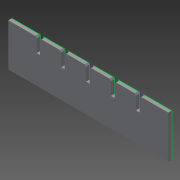
# Autodesk Inventor part: SlotRuler
Saved by Autodesk Inventor 2015 (Build 190159000, 159)
## iProperties
Created: 2015-02-15
Part Number: SlotRuler
Material: Generic
Document SubType Name: Modeling
Designer: Iain
Density: 1 g/cm^3
Appearance: Default
Author: Iain
Autodesk Inventor part; units mm, degrees
ref_plane "YZ Plane" through (0, 0, 0) normal (1, 0, 0) x (0, 1, 0)
ref_plane "XZ Plane" through (0, 0, 0) normal (0, 1, 0) x (-1, 0, 0)
ref_plane "XY Plane" through (0, 0, 0) normal (0, 0, 1) x (1, 0, 0)
sketch "Sketch1" plane through (0, 0, 0) normal (0, 1, 0) x (-1, 0, 0)
  line L0 (75, -15) -> (-75, -15)
  line L1 (-75, -15) -> (-75, 15)
  line L2 (-75, 15) -> (75, 15)
  line L3 (75, 15) -> (75, -15)
  point P0 (0, 0)
  point P1 (0, -15)
  point P2 (75, 0)
  point P3 (0, 15)
  dimension "d0" = 150
  dimension "d1" = 30
  constraints: 8 end point, 3 midpoint, 2 parallel, 1 horizontal, 1 horizontal alignment, 1 perpendicular, 1 vertical alignment
  measures "d0" distance of L1.end L2.end
  measures "d1" distance of L2.end L0.start
extrude "Extrusion1" add sketch "Sketch1" along normal blind 2.5
sketch "Sketch3" plane through (0, 2.5, 0) normal (0, 1, 0) x (1, 0, 0)
  line L0 (-75, 15) -> (-75, -15) projected
  line L1 (-75, -15) -> (75, -15) projected
  line L2 (-55, -15) -> (-52.7, -15)
  line L3 (-52.7, -15) -> (-52.7, -5)
  line L4 (-52.7, -5) -> (-55, -5)
  line L5 (-55, -5) -> (-55, -15)
  point P0 (0, 0)
  point P1 (-53.85, -15)
  point P2 (0, -15)
  dimension "d4" = 2.3
  dimension "d5" = 10
  dimension "d6" = 20
  constraints: 8 end point, 2 midpoint, 2 parallel, 1 horizontal, 1 horizontal alignment, 1 perpendicular
  measures "d4" distance of L3.end L4.end
  measures "d5" distance of L4.end L2.start
  measures "d6" distance from line of L0 L4.end
extrude "-0.2" cut sketch "Sketch3" along normal through all both and the other way through all
sketch "Sketch4" plane through (0, 2.5, 0) normal (0, 1, 0) x (1, 0, 0)
  line L0 (-75, -15) -> (-55, -15) projected
  line L1 (-37.7, -5) -> (-35.3, -5)
  line L2 (-35.3, -5) -> (-35.3, -15)
  line L3 (-35.3, -15) -> (-37.7, -15)
  line L4 (-37.7, -15) -> (-37.7, -5)
  point P0 (-52.7, -15)
  point P1 (0, 0)
  point P2 (-36.5, -15)
  point P3 (-65, -15)
  dimension "d9" = 10
  dimension "d10" = 2.4
  dimension "d11" = 15
  constraints: 8 end point, 2 midpoint, 2 parallel, 1 horizontal, 1 horizontal alignment, 1 perpendicular
  measures "d9" distance of L3.end L1.start
  measures "d10" distance of L1.start L1.end
  measures "d11" distance of point (-52.7, -15) L3.end
extrude "-0.1" cut sketch "Sketch4" against normal through all
sketch "Sketch5" plane through (0, 2.5, 0) normal (0, 1, 0) x (1, 0, 0)
  line L0 (-75, -15) -> (-55, -15) projected
  line L1 (-20.3, -5) -> (-17.8, -5)
  line L2 (-17.8, -5) -> (-17.8, -15)
  line L3 (-17.8, -15) -> (-20.3, -15)
  line L4 (-20.3, -15) -> (-20.3, -5)
  point P0 (-35.3, -5)
  point P1 (0, 0)
  point P2 (-19.05, -15)
  point P3 (-65, -15)
  dimension "d15" = 10
  dimension "d16" = 2.5
  dimension "d17" = 15
  constraints: 8 end point, 2 midpoint, 2 parallel, 1 horizontal, 1 horizontal alignment, 1 perpendicular
  measures "d15" distance of L1.end L2.end
  measures "d16" distance of L1.start L1.end
  measures "d17" distance of point (-35.3, -5) L1.start
extrude "0.0" cut sketch "Sketch5" against normal through all
sketch "Sketch6" plane through (0, 2.5, 0) normal (0, 1, 0) x (1, 0, 0)
  line L0 (-75, -15) -> (-55, -15) projected
  line L1 (-2.8, -15) -> (-0.2, -15)
  line L2 (-0.2, -15) -> (-0.2, -5)
  line L3 (-0.2, -5) -> (-2.8, -5)
  line L4 (-2.8, -5) -> (-2.8, -15)
  point P0 (-17.8, -5)
  point P1 (0, 0)
  point P2 (-1.5, -15)
  point P3 (-65, -15)
  dimension "d20" = 10
  dimension "d21" = 2.6
  dimension "d22" = 15
  constraints: 8 end point, 2 midpoint, 2 parallel, 1 horizontal, 1 horizontal alignment, 1 perpendicular
  measures "d20" distance of L1.end L2.end
  measures "d21" distance of L2.end L3.end
  measures "d22" distance of point (-17.8, -5) L3.end
extrude "+0.1" cut sketch "Sketch6" against normal through all
sketch "Sketch7" plane through (0, 2.5, 0) normal (0, 1, 0) x (1, 0, 0)
  line L0 (-75, -15) -> (-55, -15) projected
  line L1 (14.8, -15) -> (17.5, -15)
  line L2 (17.5, -15) -> (17.5, -5)
  line L3 (17.5, -5) -> (14.8, -5)
  line L4 (14.8, -5) -> (14.8, -15)
  point P0 (-0.2, -5)
  point P1 (0, 0)
  point P2 (16.15, -15)
  point P3 (-65, -15)
  dimension "d25" = 10
  dimension "d26" = 2.7
  dimension "d27" = 15
  constraints: 8 end point, 2 midpoint, 2 parallel, 1 horizontal, 1 horizontal alignment, 1 perpendicular
  measures "d25" distance of L1.end L2.end
  measures "d26" distance of L2.end L3.end
  measures "d27" distance of point (-0.2, -5) L3.end
extrude "+0.2" cut sketch "Sketch7" against normal through all
sketch "Sketch8" plane through (0, 2.5, 0) normal (0, 1, 0) x (1, 0, 0)
  line L0 (75, 15) -> (-75, 15) projected
  line L1 (-75, 15) -> (-75, -15) projected
  line L2 (-75, -15) -> (-55, -15) projected
  line L3 (-75, 15) -> (37.5, 15)
  line L4 (37.5, 15) -> (37.5, -15)
  line L5 (37.5, -15) -> (-75, -15)
  line L6 (-75, -15) -> (-75, 15)
  point P0 (17.5, -5)
  point P1 (0, 0)
  point P2 (-18.75, -15)
  point P3 (-65, -15)
  point P4 (-18.75, 15)
  point P5 (0, 15)
  point P6 (-75, 0)
  point P7 (-75, 0)
  dimension "d30" = 20
  constraints: 8 end point, 6 midpoint, 2 horizontal alignment, 2 parallel, 1 coincident, 1 horizontal, 1 perpendicular
  measures "d30" distance from line of L4 point (17.5, -5)
extrude "Extrusion7" cut sketch "Sketch8" against normal through all keep common part
sketch "Sketch9" plane through (0, 2.5, 0) normal (0, 1, 0) x (1, 0, 0)
  line L0 (37.5, 15) -> (37.5, -15) projected
  line L1 (37.5, 15) -> (-75, 15) projected
  line L2 (-75, 15) -> (-75, -15) projected
  line L3 (-75, -15) -> (-55, -15) projected
  line L4 (-55, -15) -> (-55, -5) projected
  line L5 (-55, -5) -> (-52.7, -5) projected
  line L6 (-52.7, -5) -> (-52.7, -15) projected
  line L7 (-52.7, -15) -> (-37.7, -15) projected
  line L8 (-37.7, -15) -> (-37.7, -5) projected
  line L9 (-37.7, -5) -> (-35.3, -5) projected
  line L10 (-35.3, -5) -> (-35.3, -15) projected
  line L11 (-35.3, -15) -> (-20.3, -15) projected
  line L12 (-20.3, -15) -> (-20.3, -5) projected
  line L13 (-20.3, -5) -> (-17.8, -5) projected
  line L14 (-17.8, -5) -> (-17.8, -15) projected
  line L15 (-17.8, -15) -> (-2.8, -15) projected
  line L16 (-2.8, -15) -> (-2.8, -5) projected
  line L17 (-2.8, -5) -> (-0.2, -5) projected
  line L18 (-0.2, -5) -> (-0.2, -15) projected
  line L19 (-0.2, -15) -> (14.8, -15) projected
  line L20 (14.8, -15) -> (14.8, -5) projected
  line L21 (14.8, -5) -> (17.5, -5) projected
  line L22 (17.5, -5) -> (17.5, -15) projected
  line L23 (17.5, -15) -> (37.5, -15) projected
  line L24 (-59.8913, 6.3499) -> (-47.8087, 6.3499) construction
  line L25 (-47.8087, 6.3499) -> (-47.8087, 1.1392) construction
  line L26 (-47.8087, 1.1392) -> (-59.8913, 1.1392) construction
  line L27 (-59.8913, 1.1392) -> (-59.8913, 6.3499) construction
  line L28 (-42.3413, 6.3478) -> (-30.6587, 6.3478) construction
  line L29 (-30.6587, 6.3478) -> (-30.6587, 1.1412) construction
  line L30 (-30.6587, 1.1412) -> (-42.3413, 1.1412) construction
  line L31 (-42.3413, 1.1412) -> (-42.3413, 6.3478) construction
  line L32 (-23.8434, 6.3478) -> (-14.2566, 6.3478) construction
  line L33 (-14.2566, 6.3478) -> (-14.2566, 1.1412) construction
  line L34 (-14.2566, 1.1412) -> (-23.8434, 1.1412) construction
  line L35 (-23.8434, 1.1412) -> (-23.8434, 6.3478) construction
  line L36 (8.8546, 6.3499) -> (23.4454, 6.3499) construction
  line L37 (23.4454, 6.3499) -> (23.4454, 1.1392) construction
  line L38 (23.4454, 1.1392) -> (8.8546, 1.1392) construction
  line L39 (8.8546, 1.1392) -> (8.8546, 6.3499) construction
  line L40 (-8.5954, 6.3478) -> (5.5954, 6.3478) construction
  line L41 (5.5954, 6.3478) -> (5.5954, 1.1412) construction
  line L42 (5.5954, 1.1412) -> (-8.5954, 1.1412) construction
  line L43 (-8.5954, 1.1412) -> (-8.5954, 6.3478) construction
  point P0 (0, 0)
  point P1 (-53.85, 1.1392)
  point P2 (-53.85, -5)
  point P3 (-36.5, 1.1412)
  point P4 (-36.5, -5)
  point P5 (-19.05, 1.1412)
  point P6 (-19.05, -5)
  point P7 (-1.5, -5)
  point P8 (16.15, 1.1392)
  point P9 (16.15, -5)
  point P10 (-47.8087, 3.7445)
  point P11 (-42.3413, 3.7445)
  point P12 (-30.6587, 3.7445)
  point P13 (-23.8434, 3.7445)
  point P14 (-1.5, 1.1412)
  point P15 (-1.5, -5)
  point P16 (-14.2566, 3.7445)
  point P17 (-8.5954, 3.7445)
  point P18 (5.5954, 3.7445)
  point P19 (8.8546, 3.7445)
  constraints: 19 midpoint, 5 vertical alignment, 4 horizontal alignment, 10 other
chamfer "Chamfer1" distance 1 angle 45 10 edges at (-55, 1.25, 15) (-52.7, 1.25, 15) (-37.7, 1.25, 15) (-35.3, 1.25, 15) (-20.3, 1.25, 15) (-17.8, 1.25, 15) (-2.8, 1.25, 15) (-0.2, 1.25, 15) (14.8, 1.25, 15) (17.5, 1.25, 15)
equation "\"d2\" = CardThickness"
equation "\"d12\" = CardThickness"
equation "\"d16\" = CardThickness"
equation "\"d18\" = CardThickness"
equation "\"d23\" = CardThickness"
equation "\"d28\" = CardThickness"
equation "\"d31\" = CardThickness"
equation "\"CardThickness\" = 2.5"
body "Solid1"
